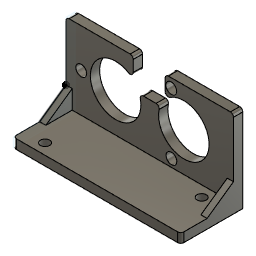
ultrasonic_support v5 (Autodesk Fusion 360 design; units mm, degrees)
Autodesk Fusion 360 part; units mm, degrees
sketch "Sketch1" plane through (0, 0, 0) normal (0, 1, 0) x (1, 0, 0)
  line L0 (0, 0) -> (-54, 0)
  line L1 (-54, 0) -> (-54, -20)
  line L2 (-54, -20) -> (0, -20)
  line L3 (0, -20) -> (0, 0)
  dimension "d5" = 54
  dimension "d6" = 20
  constraint horizontal L0
  constraint vertical L1
  constraint horizontal L2
  constraint vertical L3
  constraint coincident L0.start L3.end
  measures "d5" distance of L0.start L0.end
  measures "d6" distance of L0.end L1.end
extrude "Extrude1" add sketch "Sketch1" along normal blind 3
sketch "Sketch2" plane through (0, 3, 0) normal (0, 1, 0) x (-1, 0, 0)
  line L0 (0, 20) -> (0, 0)
  line L1 (0, 0) -> (54, 0)
  line L2 (54, 0) -> (54, 20)
  line L3 (54, 20) -> (0, 20)
  line L4 (0, 0) -> (54, 0)
  line L5 (54, 0) -> (54, 3)
  line L6 (54, 3) -> (0, 3)
  line L7 (0, 3) -> (0, 0)
  dimension "d9" = 3
  constraint horizontal L4
  constraint vertical L5
  constraint horizontal L6
  constraint vertical L7
  constraint coincident L2 L5.end
  constraint coincident L0.end L1.start
  measures "d9" distance of L1.end L5.end
extrude "Extrude2" add sketch "Sketch2" along normal blind 25 contours L0 L1 L2 L4 L5 L6 L7
sketch "Sketch3" plane through (0, 3, 0) normal (0, 1, 0) x (-1, 0, 0)
  line L0 (0, 3) -> (54, 3)
  line L1 (54, 3) -> (54, 20)
  line L2 (54, 20) -> (0, 20)
  line L3 (0, 20) -> (0, 3)
  circle A0 centre (6.75, 6.5) radius 1.5
  circle A1 centre (47.25, 16.5) radius 1.5
  line L4 (6.75, 16.5) -> (47.25, 16.5) construction
  line L5 (47.25, 16.5) -> (47.25, 6.5) construction
  line L6 (47.25, 6.5) -> (6.75, 6.5) construction
  line L7 (6.75, 6.5) -> (6.75, 16.5) construction
  line L8 (6.75, 16.5) -> (47.25, 6.5) construction
  line L9 (47.25, 16.5) -> (6.75, 6.5) construction
  line L10 (0, 20) -> (54, 3) construction
  line L11 (54, 20) -> (0, 3) construction
  point P0 (27, 11.5)
  point P1 (27, 11.5)
  dimension "d12" = 10
  dimension "d13" = 40.5
  dimension "d16" = 3
  dimension "d17" = 3
  constraint horizontal L4
  constraint vertical L5
  constraint horizontal L6
  constraint vertical L7
  constraint coincident A0.centre L6.end
  constraint coincident A1.centre L4.end
  constraint midpoint L9 P1
  constraint coincident L2.end L3.start
  constraint coincident L0.end L1.start
  constraint coincident L1.end L2.start
  constraint coincident L0.start L3.end
  constraint midpoint L11 P1
  constraint coincident P1 P0
  measures "d12" distance of L4.start A0.centre
  measures "d13" distance of L4.start A1.centre
  measures "d16" diameter of A0
  measures "d17" diameter of A1
extrude "Extrude3" cut sketch "Sketch3" against normal up to surface (3 mm away) contours A0 | A1
sketch "Sketch4" plane through (0, 0, 0) normal (0, 0, -1) x (-1, 0, 0)
  line L0 (0, 0) -> (54, 0)
  line L1 (54, 0) -> (54, 28)
  line L2 (54, 28) -> (0, 28)
  line L3 (0, 28) -> (0, 0)
  line L4 (2, 28) -> (52, 28) construction
  line L5 (52, 28) -> (52, 3) construction
  line L6 (52, 3) -> (2, 3) construction
  line L7 (2, 3) -> (2, 28) construction
  circle A0 centre (20, 5.5) radius 1.75
  circle A1 centre (49.085, 15.5) radius 1.75
  line L8 (2, 15.5) -> (52, 15.5) construction
  line L9 (22.016, 28) -> (32.316, 28)
  line L10 (32.316, 28) -> (32.316, 21.3408)
  line L11 (30.3834, 18.4) -> (23.6166, 18.4)
  line L12 (22.016, 20.9982) -> (22.016, 28)
  circle A2 centre (20.062, 25.085) radius 1.75
  arc A3 (22.016, 20.9982) -> (23.6166, 18.4) centre (16, 15.5) ccw
  arc A4 (30.3834, 18.4) -> (32.316, 21.3408) centre (38, 15.5) ccw
  point P0 (27, 28)
  dimension "d20" = 50
  dimension "d21" = 25
  dimension "d24" = 18
  dimension "d25" = 2.5
  dimension "d26" = 3.5
  dimension "d27" = 3.5
  dimension "d28" = 2.915
  dimension "d29" = 12.5
  dimension "d30" = 16.3
  dimension "d31" = 16.3
  dimension "d33" = 14
  dimension "d34" = 14
  dimension "d35" = 20.016
  dimension "d36" = 9.6
  dimension "d37" = 3.5
  dimension "d38" = 2.915
  dimension "d39" = 18.062
  dimension "d40" = 10.3
  constraint horizontal L4
  constraint vertical L5
  constraint horizontal L6
  constraint vertical L7
  constraint collinear L2 L4
  constraint coincident L4 P0
  constraint midpoint L4 P0
  constraint midpoint L2 P0
  constraint coincident L5 L8.end
  constraint perpendicular L5 L8
  constraint midpoint L7 L8.start
  constraint coincident A4.centre L8
  constraint coincident A3.centre L8
  constraint horizontal L9
  constraint vertical L10
  constraint horizontal L11
  constraint vertical L12
  constraint coincident L4 L9.start
  measures "d20" distance of L4.start L4.end
  measures "d21" distance of L4.start L6.end
  measures "d24" distance of L7 A0.centre
  measures "d25" distance of L6 A0.centre
  measures "d26" diameter of A0
  measures "d27" diameter of A1
  measures "d28" distance of L5 A1.centre
  measures "d29" distance of L6 A1.centre
  measures "d30" diameter of A4
  measures "d31" diameter of A3
  measures "d33" distance of L5 A4.centre
  measures "d34" distance of L7 A3.centre
  measures "d35" distance of L7 L12
  measures "d36" distance of L4 L11
  measures "d37" diameter of A2
  measures "d38" distance of L4 A2.centre
  measures "d39" distance of L7 A2.centre
  measures "d40" distance of L10 L12
extrude "Extrude4" cut sketch "Sketch4" against normal up to surface (3 mm away) contours L2 L9 L10 L11 L12 A3 A4 | A0 | A1 | A2
sketch "Sketch5" plane through (-54, 0, 0) normal (-1, 0, 0) x (0, 0, 1)
  line L0 (0, 0) -> (20, 0)
  line L1 (20, 0) -> (20, 3)
  line L2 (20, 3) -> (3, 3)
  line L3 (3, 3) -> (3, 28)
  line L4 (3, 28) -> (0, 28)
  line L5 (0, 28) -> (0, 0)
  line L6 (3, 9) -> (11.5, 3)
  dimension "d46" = 6
  constraint midpoint L2 L6.end
  constraint coincident L3 L6.start
  measures "d46" distance of L2.end L6.start
extrude "Extrude5" add sketch "Sketch5" against normal blind 2 contours L2 L3 L6
ref_plane "WorkPlane1" through (-27, 14, 10) normal (-1, 0, 0) x (0, 0, 1)
fillet "Fillet1" radius 1 10 edges at (-54, 28, 1.5) (-54, 1.5, 20) (-32.316, 28, 1.5) (-32.316, 21.3408, 1.5) (-30.3834, 18.4, 1.5) (-23.6166, 18.4, 1.5) (-22.016, 20.9982, 1.5) (-22.016, 28, 1.5) (0, 28, 1.5) (0, 1.5, 20)
mirror "Mirror1" about plane through (-27, 14, 10) normal (-1, 0, 0) of "Extrude5"
equation "height_base = 20 mm"
equation "width = 54 mm"
equation "thick = 3 mm"
equation "height_sensor = 25 mm"
equation "d5 = width"
equation "d6 = height_base"
equation "d7 = thick"
equation "d9 = thick"
equation "d10 = height_sensor"
equation "d12 = height_base * 1 / 2"
equation "d13 = width * 3 / 4"
equation "screw_base = 3 mm"
equation "screw_sensor = 3.5 mm"
equation "d16 = screw_base"
equation "d17 = screw_base"
equation "d26 = screw_sensor"
equation "d27 = screw_sensor"
equation "d30 = sensor"
equation "d31 = sensor"
equation "sensor = 16.3 mm"
equation "d37 = screw_sensor"
equation "fillet = 1 mm"
equation "d51 = fillet"
